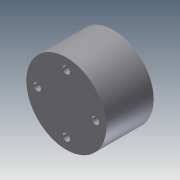
# Autodesk Inventor part: awesomespin
Saved by Autodesk Inventor 2011 (Build 150239000, 239)
## iProperties
Created: 2011-12-10
Part Number: awesomespin
Document SubType Name: Modeling
Designer: Matthew
Density: 1 g/cm^3
Author: Matthew
Autodesk Inventor part; units mm, degrees
ref_plane "YZ Plane" through (0, 0, 0) normal (1, 0, 0) x (0, 1, 0)
ref_plane "XZ Plane" through (0, 0, 0) normal (0, 1, 0) x (-1, 0, 0)
ref_plane "XY Plane" through (0, 0, 0) normal (0, 0, 1) x (1, 0, 0)
sketch "Sketch1" plane through (0, 0, 0) normal (0, 0, 1) x (1, 0, 0)
  circle A0 centre (0, 0) radius 11
  dimension "d0" = 22
  constraints: 1 centre point, 1 coincident
  measures "d0" diameter of A0
extrude "Extrusion1" add sketch "Sketch1" along normal blind 10
sketch "Sketch2" plane through (0, 0, 10) normal (0, 0, 1) x (1, 0, 0)
  circle A0 centre (0, 0) radius 11 projected
  circle A1 centre (0, 0) radius 8
  circle A2 centre (-8, 0) radius 1
  circle A3 centre (0, 8) radius 1
  circle A4 centre (8, 0) radius 1
  circle A5 centre (0, -8) radius 1
  dimension "d3" = 16
  dimension "d4" = 2
  dimension "d5" = 2
  dimension "d6" = 2
  dimension "d7" = 2
  constraints: 5 centre point, 4 point on circle, 1 coincident
  measures "d3" diameter of A1
  measures "d4" diameter of A2
  measures "d5" diameter of A3
  measures "d6" diameter of A4
  measures "d7" diameter of A5
extrude "Extrusion2" cut sketch "Sketch2" against normal blind 10 contours A1 A4 | A1 A4 | A3 A1 | A1 A3 | A5 A1 | A1 A5 | A2 A1 | A1 A2
sketch "Sketch3" plane through (0, 0, 10) normal (0, 0, 1) x (1, 0, 0)
  circle A0 centre (8, 0) radius 1 projected
  circle A1 centre (0, -8) radius 1 projected
  circle A2 centre (-8, 0) radius 1 projected
  circle A3 centre (0, 8) radius 1 projected
  circle A4 centre (0, 0) radius 11 projected
extrude "Extrusion3" add sketch "Sketch3" along normal blind 3
body "Solid1"
